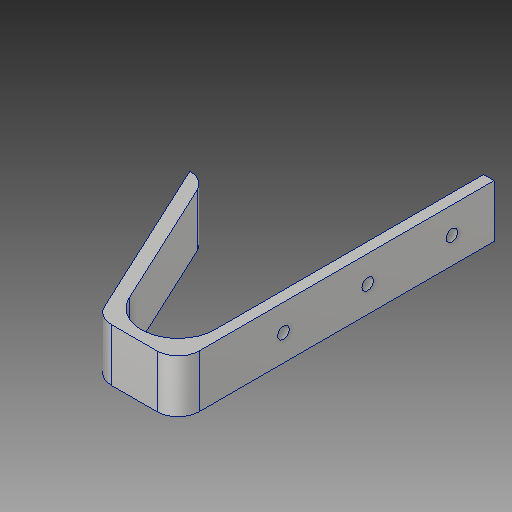
# Autodesk Inventor part: Hook
Saved by Autodesk Inventor 2019.4 (Build 234330000, 330)
## iProperties
Created: 2020-01-11
Part Number: Hook
Material: Aluminum 6061
Document SubType Name: Modeling
Designer: Mark
Density: 2.7 g/cm^3
Appearance: Aluminum - Flat
Mass: 99.2212 g
Surface Area: 163.544 cm^2
Volume: 36.7486 cm^3
Author: Mark
Autodesk Inventor part; units mm, degrees
ref_plane "YZ Plane" through (0, 0, 0) normal (1, 0, 0) x (0, 1, 0)
ref_plane "XZ Plane" through (0, 0, 0) normal (0, 1, 0) x (-1, 0, 0)
ref_plane "XY Plane" through (0, 0, 0) normal (0, 0, 1) x (1, 0, 0)
sketch "Sketch1" plane through (0, 0, 0) normal (0, 1, 0) x (-1, 0, 0)
  line L0 (-2.5, -75) -> (2.5, -75)
  line L1 (2.5, -75) -> (2.5, 75)
  line L2 (2.5, 75) -> (-2.5, 75)
  line L3 (-2.5, 75) -> (-2.5, -75)
  line L4 (-2.5, -75) -> (2.5, 75) construction
  line L5 (2.5, -75) -> (-2.5, 75) construction
  line L6 (2.5, 75) -> (35.5, 75)
  line L7 (35.5, 75) -> (35.5, 35)
  line L8 (35.5, 35) -> (2.5, 35)
  line L9 (2.5, 35) -> (2.5, 75)
  line L10 (35.5, 75) -> (73.5356, -6.5677)
  line L11 (35.5, 75) -> (125.5, 75) construction
  line L12 (73.5356, -6.5677) -> (2.5, -6.5677)
  line L13 (73.5356, -6.5677) -> (144.5713, -6.5677) construction
  point P0 (0, 0)
  dimension "d0" = 5
  dimension "d1" = 150
  dimension "d2" = 33
  dimension "d3" = 40
  dimension "d4" = 90
  dimension "d5" = 65
  dimension "d6" = 180
  constraints: 28 end point, 4 horizontal, 4 parallel, 2 equal length, 2 midpoint, 2 perpendicular, 1 point on line
  measures "d0" distance of L2.end L1.end
  measures "d1" distance of L1.end L0.end
  measures "d2" distance of L7.end L8.end
  measures "d3" distance of L6.end L7.end
  measures "d4" distance of L6.end L10.end
  measures "d5" angle of L10 L11
  measures "d6" angle of L12 L13
extrude "Extrusion1" add sketch "Sketch1" along normal blind 25
sketch "Sketch2" plane through (0, 0, 0) normal (0, -1, 0) x (1, 0, 0)
  circle A0 centre (-20, 52.5) radius 17.5
  line L0 (2.5, -75) -> (2.5, 75) projected
  line L1 (2.5, 75) -> (-35.5, 75) projected
  line L2 (-66.8528, -6.5677) -> (-35.8604, 59.8958)
  line L3 (-35.5, 75) -> (-73.5356, -6.5677) projected
  line L4 (-2.5, 52.5) -> (-2.5, -6.5677)
  line L5 (-2.5, -6.5677) -> (-73.5356, -6.5677) projected
  line L6 (-2.5, 52.5) -> (56.5677, 52.5) construction
  line L7 (-66.8528, -6.5677) -> (-2.5, -6.5677)
  line L8 (-73.5356, -6.5677) -> (-2.5, -6.5677) projected
  point P0 (0, 0)
  dimension "d9" = 35
  dimension "d10" = 22.5
  dimension "d11" = 22.5
  dimension "d12" = 90
  constraints: 8 end point, 2 point on circle, 2 point on line, 2 tangent, 1 centre point, 1 horizontal, 1 parallel, 1 perpendicular
  measures "d9" diameter of A0
  measures "d10" distance from line of L0 A0.centre
  measures "d11" distance from line of L1 A0.centre
  measures "d12" angle of L4 L6
extrude "Extrusion2" cut sketch "Sketch2" against normal blind 25
fillet "Fillet1" radius 10 3 edges at (-35.5, 12.5, 75) (2.5, 12.5, 75) (-66.8528, 12.5, -6.5677)
sketch "Sketch3" plane through (-2.5, 0, -75) normal (-1, 0, 0) x (0, 0, 1)
  circle A0 centre (20, 12.5) radius 2.75
  circle A1 centre (60, 12.5) radius 2.75
  circle A2 centre (100, 12.5) radius 2.75
  line L0 (0, 25) -> (127.5, 25) projected
  line L1 (0, 0) -> (0, 25) projected
  point P0 (75, 0)
  dimension "d16" = 5.5
  dimension "d17" = 5.5
  dimension "d18" = 5.5
  dimension "d19" = 12.5
  dimension "d20" = 12.5
  dimension "d21" = 12.5
  dimension "d22" = 20
  dimension "d23" = 40
  dimension "d24" = 40
  constraints: 3 centre point
  measures "d16" diameter of A0
  measures "d17" diameter of A1
  measures "d18" diameter of A2
  measures "d19" distance from line of L0 A2.centre
  measures "d20" distance from line of L0 A1.centre
  measures "d21" distance from line of L0 A0.centre
  measures "d22" distance from line of L1 A0.centre
  measures "d23" distance of A0.centre A1.centre
  measures "d24" distance of A1.centre A2.centre
extrude "Extrusion3" cut sketch "Sketch3" against normal blind 25
body "Solid1"
